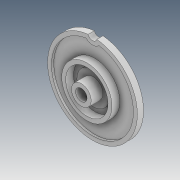
# Autodesk Inventor part: PMSealNoAxle
Saved by Autodesk Inventor 2020 (Build 240168000, 168)
## iProperties
Created: 2020-05-07
Part Number: PMSealNoAxle
Material: Generic
Document SubType Name: Modeling
Designer: Theo Cominotto
Density: 1 g/cm^3
Appearance: Default
Author: Theo Cominotto
Autodesk Inventor part; units mm, degrees
ref_plane "YZ Plane" through (0, 0, 0) normal (1, 0, 0) x (0, 1, 0)
sketch "Sketch1" plane through (0, 0, 0) normal (0, 0, 1) x (1, 0, 0)
  circle A0 centre (0, 0) radius 11.4
  dimension "d0" = 22.8
  constraints: 1 centre point, 1 coincident
  measures "d0" diameter of A0
extrude "Extrusion1" add sketch "Sketch1" along normal blind 1
ref_plane "Work Plane1" through (0, 0, 1) normal (0, 0, 1) x (1, 0, 0)
sketch "Sketch3" plane through (0, 0, 1) normal (0, 0, 1) x (1, 0, 0)
  circle A0 centre (0, 0) radius 6.375
  circle A1 centre (0, 0) radius 5.375
  dimension "d6" = 12.75
  dimension "d7" = 10.75
  constraints: 2 centre point, 2 coincident
  measures "d6" diameter of A0
  measures "d7" diameter of A1
extrude "Extrusion3" add sketch "Sketch3" along normal blind 2
ref_plane "Work Plane2" through (0, 0, 1) normal (0, 0, 1) x (1, 0, 0)
sketch "Sketch5" plane through (0, 0, 1) normal (0, 0, 1) x (1, 0, 0)
  circle A0 centre (0, 0) radius 4.125
  dimension "d14" = 8.25
  constraints: 1 centre point, 1 coincident
  measures "d14" diameter of A0
extrude "Extrusion5" add sketch "Sketch5" along normal blind 0.4
sketch "Sketch6" plane through (0, 0, 0) normal (0, 0, -1) x (-1, 0, 0)
  circle A0 centre (0, 0) radius 1.45
  dimension "d17" = 2.9
  constraints: 1 centre point, 1 coincident
  measures "d17" diameter of A0
extrude "Extrusion6" cut sketch "Sketch6" against normal up to surface (1.4 mm away)
sketch "Sketch7" plane through (0, 0, 1.4) normal (0, 0, 1) x (1, 0, 0)
  circle A0 centre (0, 0) radius 1.45 projected
  circle A1 centre (0, 0) radius 1.45 projected
  circle A2 centre (0, 0) radius 2.5
  dimension "d20" = 5
  constraints: 1 centre point, 1 coincident
  measures "d20" diameter of A2
extrude "Pressguide" add sketch "Sketch7" along normal blind 3
sketch "Sketch8" plane through (0, 0, 1) normal (0, 0, 1) x (1, 0, 0)
  circle A0 centre (0, 0) radius 11.4 projected
  line L0 (-1.1, 11.3468) -> (1.1, 11.3468) construction
  line L1 (0, 11.3468) -> (0, 10.5468) construction
  arc A1 (-1.1, 11.3468) -> (1.1, 11.3468) centre (0, 11.7031) ccw
  dimension "d23" = 2.2
  dimension "d24" = 0.8
  constraints: 5 point on circle, 4 end point, 1 centre point, 1 horizontal, 1 midpoint, 1 vertical
  measures "d23" distance of L0.start L0.end
  measures "d24" distance of L1.start L1.end
extrude "Extrusion8" cut sketch "Sketch8" against normal up to surface (1 mm away) contours A1 A0 picked at (-0.044, 11.1142)
sketch "Sketch9" plane through (0, 0, 1) normal (0, 0, 1) x (1, 0, 0)
  arc A0 (-1.1, 11.3468) -> (1.1, 11.3468) centre (0, 0) ccw projected
  arc A1 (-1.1, 11.3468) -> (1.1, 11.3468) centre (0, 11.7031) ccw projected
  arc A2 (-1.6146, 10.2739) -> (1.6146, 10.2739) centre (0, 0) ccw
  arc A3 (-1.6146, 10.2739) -> (1.6146, 10.2739) centre (0, 11.7031) ccw
  dimension "d27" = 1
  constraints: 4 point on circle, 2 centre point, 1 other
  measures "d27" radial gap between concentric circles of A0 A2
extrude "Extrusion9" add sketch "Sketch9" along normal blind 0.57
sketch "Sketch10" plane through (0, 0, 0) normal (0, 0, -1) x (-1, 0, 0)
  circle A0 centre (0, 0) radius 1.45 projected
extrude "Axle" [suppressed]
body "Solid1"
